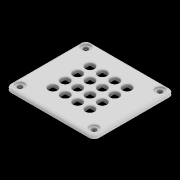
# Autodesk Inventor part: Cubierta Botonera Redonda
Saved by Autodesk Inventor 2020 (Build 240168000, 168)
## iProperties
Created: 2022-02-20
Part Number: Cubierta Botonera Redonda
Material: Genérico
Document SubType Name: Modeling
Designer: Alférez
Density: 1 g/cm^3
Appearance: Valor por defecto
Author: Alférez
Autodesk Inventor part; units mm, degrees
ref_plane "YZ Plane" through (0, 0, 0) normal (1, 0, 0) x (0, 1, 0)
ref_plane "XZ Plane" through (0, 0, 0) normal (0, 1, 0) x (-1, 0, 0)
ref_plane "XY Plane" through (0, 0, 0) normal (0, 0, 1) x (1, 0, 0)
sketch "Boceto1" plane through (0, 0, 0) normal (0, 1, 0) x (-1, 0, 0)
  line L0 (0, 0) -> (90, 0)
  line L1 (90, 0) -> (90, -80)
  line L2 (90, -80) -> (0, -80)
  line L3 (0, -80) -> (0, 0)
  line L4 (0, 0) -> (17, 0)
  line L5 (17, 0) -> (17, -12)
  line L6 (17, -12) -> (28, -12)
  line L7 (28, -12) -> (28, -23)
  line L8 (28, -23) -> (17, -23)
  line L9 (17, -23) -> (17, -12)
  line L10 (17, -23) -> (17, -27)
  line L11 (17, -27) -> (28, -27)
  line L12 (28, -27) -> (28, -38)
  line L13 (28, -38) -> (17, -38)
  line L14 (17, -38) -> (17, -27)
  line L15 (17, -38) -> (17, -42)
  line L16 (17, -42) -> (28, -42)
  line L17 (28, -42) -> (28, -53)
  line L18 (28, -53) -> (17, -53)
  line L19 (17, -53) -> (17, -42)
  line L20 (17, -53) -> (17, -57)
  line L21 (17, -57) -> (28, -57)
  line L22 (28, -57) -> (28, -68)
  line L23 (28, -68) -> (17, -68)
  line L24 (17, -68) -> (17, -57)
  line L25 (32, -12) -> (43, -12)
  line L26 (43, -12) -> (43, -23)
  line L27 (43, -23) -> (32, -23)
  line L28 (32, -23) -> (32, -12)
  line L29 (32, -23) -> (32, -27)
  line L30 (32, -27) -> (43, -27)
  line L31 (43, -27) -> (43, -38)
  line L32 (43, -38) -> (32, -38)
  line L33 (32, -38) -> (32, -27)
  line L34 (32, -38) -> (32, -42)
  line L35 (32, -42) -> (43, -42)
  line L36 (43, -42) -> (43, -53)
  line L37 (43, -53) -> (32, -53)
  line L38 (32, -53) -> (32, -42)
  line L39 (32, -53) -> (32, -57)
  line L40 (32, -57) -> (43, -57)
  line L41 (43, -57) -> (43, -68)
  line L42 (43, -68) -> (32, -68)
  line L43 (32, -68) -> (32, -57)
  line L44 (43, -12) -> (47, -12)
  line L45 (47, -12) -> (58, -12)
  line L46 (58, -12) -> (58, -23)
  line L47 (58, -23) -> (47, -23)
  line L48 (47, -23) -> (47, -12)
  line L49 (47, -23) -> (47, -27)
  line L50 (47, -27) -> (58, -27)
  line L51 (58, -27) -> (58, -38)
  line L52 (58, -38) -> (47, -38)
  line L53 (47, -38) -> (47, -27)
  line L54 (47, -38) -> (47, -42)
  line L55 (47, -42) -> (58, -42)
  line L56 (58, -42) -> (58, -53)
  line L57 (58, -53) -> (47, -53)
  line L58 (47, -53) -> (47, -42)
  line L59 (47, -53) -> (47, -57)
  line L60 (47, -57) -> (58, -57)
  line L61 (58, -57) -> (58, -68)
  line L62 (58, -68) -> (47, -68)
  line L63 (47, -68) -> (47, -57)
  line L64 (58, -12) -> (62, -12)
  line L65 (73, -23) -> (62, -23)
  line L66 (62, -23) -> (62, -27)
  line L67 (62, -27) -> (73, -27)
  line L68 (73, -12) -> (73, -23)
  line L69 (62, -23) -> (62, -12)
  line L70 (62, -38) -> (62, -27)
  line L71 (62, -38) -> (62, -42)
  line L72 (73, -38) -> (62, -38)
  line L73 (73, -27) -> (73, -38)
  line L74 (62, -12) -> (73, -12)
  line L75 (62, -42) -> (73, -42)
  line L76 (62, -53) -> (62, -42)
  line L77 (73, -42) -> (73, -53)
  line L78 (62, -53) -> (62, -57)
  line L79 (62, -57) -> (73, -57)
  line L80 (62, -68) -> (62, -57)
  line L81 (73, -57) -> (73, -68)
  line L82 (73, -68) -> (62, -68)
  line L83 (73, -53) -> (62, -53)
  line L84 (28, -12) -> (32, -12)
  line L85 (0, 0) -> (8.5, 0)
  line L86 (0, 8.5) -> (0, 0)
  line L87 (0, 0) -> (-8.5, 0)
  line L88 (0, -8.5) -> (0, 0)
  line L89 (0, -80) -> (8.5, -80)
  line L90 (0, -88.5) -> (0, -80)
  line L91 (0, -80) -> (-8.5, -80)
  line L92 (0, -71.5) -> (0, -80)
  line L93 (90, 0) -> (81.5, 0)
  line L94 (90, 8.5) -> (90, 0)
  line L95 (90, 0) -> (98.5, 0)
  line L96 (90, -8.5) -> (90, 0)
  line L97 (90, -80) -> (81.5, -80)
  line L98 (81.5, -80) -> (81.5, -71.5)
  line L99 (90, -80) -> (98.5, -80)
  line L100 (90, -71.5) -> (90, -80)
  circle A0 centre (90, 0) radius 3
  circle A1 centre (90, -80) radius 3
  circle A2 centre (0, 0) radius 3
  circle A3 centre (0, -80) radius 3
  line L101 (0, 0) -> (-8.5, 0)
  line L102 (-8.5, 0) -> (-8.5, 8.5)
  line L103 (-8.5, 8.5) -> (0, 8.5)
  line L104 (0, 8.5) -> (0, 0)
  line L105 (0, -88.5) -> (-8.5, -88.5)
  line L106 (-8.5, -88.5) -> (-8.5, -80)
  line L107 (-8.5, -80) -> (0, -80)
  line L108 (0, -80) -> (0, -88.5)
  line L109 (98.5, 0) -> (90, 0)
  line L110 (90, 0) -> (90, 8.5)
  line L111 (90, 8.5) -> (98.5, 8.5)
  line L112 (98.5, 8.5) -> (98.5, 0)
  line L113 (98.5, -88.5) -> (90, -88.5)
  line L114 (90, -88.5) -> (90, -80)
  line L115 (90, -80) -> (98.5, -80)
  line L116 (98.5, -80) -> (98.5, -88.5)
  line L117 (98.5, 8.5) -> (-8.5, 8.5)
  line L118 (-8.5, 8.5) -> (-8.5, -88.5)
  line L119 (-8.5, -88.5) -> (98.5, -88.5)
  line L120 (98.5, -88.5) -> (98.5, 8.5)
  dimension "d0" = 90
  dimension "d1" = 80
  dimension "d2" = 17
  dimension "d3" = 12
  dimension "d4" = 11
  dimension "d5" = 11
  dimension "d6" = 4
  dimension "d7" = 11
  dimension "d8" = 11
  dimension "d9" = 4
  dimension "d10" = 11
  dimension "d11" = 11
  dimension "d12" = 4
  dimension "d13" = 11
  dimension "d14" = 11
  dimension "d16" = 11
  dimension "d17" = 11
  dimension "d18" = 4
  dimension "d19" = 11
  dimension "d20" = 11
  dimension "d21" = 4
  dimension "d22" = 11
  dimension "d23" = 11
  dimension "d24" = 4
  dimension "d25" = 11
  dimension "d26" = 11
  dimension "d27" = 4
  dimension "d28" = 11
  dimension "d29" = 11
  dimension "d30" = 4
  dimension "d31" = 11
  dimension "d32" = 11
  dimension "d33" = 4
  dimension "d34" = 11
  dimension "d35" = 11
  dimension "d36" = 4
  dimension "d37" = 11
  dimension "d38" = 11
  dimension "d39" = 4
  dimension "d40" = 11
  dimension "d41" = 11
  dimension "d42" = 4
  dimension "d43" = 11
  dimension "d44" = 11
  dimension "d45" = 4
  dimension "d46" = 11
  dimension "d47" = 11
  dimension "d48" = 4
  dimension "d49" = 11
  dimension "d50" = 11
  dimension "d51" = 4
  dimension "d52" = 8.5
  dimension "d53" = 8.5
  dimension "d54" = 8.5
  dimension "d55" = 8.5
  dimension "d56" = 8.5
  dimension "d57" = 8.5
  dimension "d58" = 8.5
  dimension "d59" = 6
  dimension "d60" = 6
  dimension "d61" = 6
  dimension "d62" = 8.5
  dimension "d63" = 8.5
  dimension "d64" = 8.5
  constraints: 242 end point, 52 equal length, 29 horizontal, 27 perpendicular, 12 vertical, 4 centre point, 4 coincident, 1 point on line
  measures "d0" distance of L1.end L2.end
  measures "d1" distance of L0.end L1.end
  measures "d2" distance of L0.start L4.end
  measures "d3" distance of L4.end L5.end
  measures "d4" distance of L7.end L8.end
  measures "d5" distance of L6.end L7.end
  measures "d6" distance of L8.end L10.end
  measures "d7" distance of L12.end L13.end
  measures "d8" distance of L11.end L12.end
  measures "d9" distance of L13.end L15.end
  measures "d10" distance of L17.end L18.end
  measures "d11" distance of L16.end L17.end
  measures "d12" distance of L18.end L20.end
  measures "d13" distance of L22.end L23.end
  measures "d14" distance of L21.end L22.end
  measures "d16" distance of L27.start L27.end
  measures "d17" distance of L26.start L27.start
  measures "d18" distance of L27.end L29.end
  measures "d19" distance of L32.start L33.start
  measures "d20" distance of L30.end L32.start
  measures "d21" distance of L33.start L34.end
  measures "d22" distance of L36.end L38.start
  measures "d23" distance of L35.end L36.end
  measures "d24" distance of L38.start L39.end
  measures "d25" distance of L41.end L43.start
  measures "d26" distance of L40.end L41.end
  measures "d27" distance of L26.start L44.end
  measures "d28" distance of L47.start L49.start
  measures "d29" distance of L46.start L47.start
  measures "d30" distance of L49.start L53.end
  measures "d31" distance of L52.start L53.start
  measures "d32" distance of L50.end L52.start
  measures "d33" distance of L53.start L54.end
  measures "d34" distance of L57.start L58.start
  measures "d35" distance of L55.end L57.start
  measures "d36" distance of L58.start L59.end
  measures "d37" distance of L61.end L62.end
  measures "d38" distance of L60.end L61.end
  measures "d39" distance of L46.start L64.end
  measures "d40" distance of L68.end L66.start
  measures "d41" distance of L68.start L68.end
  measures "d42" distance of L66.start L66.end
  measures "d43" distance of L72.start L70.start
  measures "d44" distance of L67.end L72.start
  measures "d45" distance of L70.start L76.end
  measures "d46" distance of L83.start L78.start
  measures "d47" distance of L77.start L83.start
  measures "d48" distance of L78.start L80.end
  measures "d49" distance of L81.end L82.end
  measures "d50" distance of L81.start L81.end
  measures "d51" distance of L6.end L84.end
  measures "d52" distance of L86.end L87.end
  measures "d53" distance of L86.start L86.end
  measures "d54" distance of L91.end L90.end
  measures "d55" distance of L90.end L90.start
  measures "d56" distance of L95.end L94.end
  measures "d57" distance of L94.end L94.start
  measures "d58" distance of L99.start L99.end
  measures "d59" diameter of A0
  measures "d60" diameter of A1
  measures "d61" diameter of A2
  measures "d62" distance of L102.end L103.end
  measures "d63" distance of L101.end L102.end
  measures "d64" distance of L106.end L108.start
extrude "Extrusión1" add sketch "Boceto1" along normal blind 3 contours A2 L86 L117 L94 A0 L0 | L0 A0 L1 A1 L2 A3 L3 A2 | L3 A3 L91 L118 L87 A2 | A2 L87 L102 L103 L86 | L111 L112 L95 A0 L94 | L91 A3 L90 L105 L106 | L2 A1 L114 L119 L90 A3 | L95 L120 L99 A1 L1 A0 | L116 L113 L114 A1 L99
fillet "Empalme1" radius 6 4 edges at (-98.5, 1.5, 8.5) (-98.5, 1.5, -88.5) (8.5, 1.5, 8.5) (8.5, 1.5, -88.5)
fillet "Empalme2" radius 2 16 edges at (-96.7426, 3, -86.7426) (-98.5, 3, 1.25) (-98.5, 3, -40) (-98.5, 3, -81.25) (-96.7426, 3, 6.7426) (1.25, 3, 8.5) (-45, 3, 8.5) (-91.25, 3, 8.5) (6.7426, 3, 6.7426) (8.5, 3, 1.25) (8.5, 3, -40) (8.5, 3, -81.25) (6.7426, 3, -86.7426) (1.25, 3, -88.5) (-45, 3, -88.5) (-91.25, 3, -88.5)
fillet "Empalme3" radius 5.5 63 edges at (-73, 1.5, -12) (-58, 1.5, -12) (-43, 1.5, -12) (-28, 1.5, -12) (-28, 1.5, -27) (-43, 1.5, -27) (-58, 1.5, -27) (-73, 1.5, -27) (-73, 1.5, -42) (-73, 1.5, -57) (-58, 1.5, -42) (-58, 1.5, -57) (-43, 1.5, -57) (-43, 1.5, -42) (-28, 1.5, -42) (-28, 1.5, -57) (-73, 1.5, -23) (-73, 1.5, -38) (-73, 1.5, -68) (-73, 1.5, -53) (-58, 1.5, -68) (-58, 1.5, -53) (-58, 1.5, -38) (-43, 1.5, -38) (-43, 1.5, -68) (-43, 1.5, -53) (-43, 1.5, -23) (-58, 1.5, -23) (-28, 1.5, -23) (-28, 1.5, -38) (-28, 1.5, -53) (-28, 1.5, -68) (-62, 1.5, -68) (-47, 1.5, -68) (-32, 1.5, -68) (-17, 1.5, -68) (-17, 1.5, -53) (-32, 1.5, -53) (-47, 1.5, -53) (-32, 1.5, -38) (-47, 1.5, -38) (-62, 1.5, -38) (-17, 1.5, -38) (-17, 1.5, -23) (-32, 1.5, -23) (-47, 1.5, -23) (-62, 1.5, -23) (-17, 1.5, -57) (-17, 1.5, -42) (-17, 1.5, -27) (-17, 1.5, -12) (-32, 1.5, -12) (-32, 1.5, -27) (-32, 1.5, -42) (-32, 1.5, -57) (-47, 1.5, -27) (-47, 1.5, -12) (-47, 1.5, -42) (-47, 1.5, -57) (-62, 1.5, -57) (-62, 1.5, -42) (-62, 1.5, -27) (-62, 1.5, -12)
fillet "Empalme4" radius 5.5 1 edges at (-62, 1.5, -53)
sketch "Boceto3" plane through (0, 0, 0) normal (0, -1, 0) x (1, 0, 0)
  line L0 (-73, -12) -> (-62, -12)
  line L1 (-62, -12) -> (-62, -23)
  line L2 (-62, -23) -> (-73, -23)
  line L3 (-73, -23) -> (-73, -12)
  line L4 (-73, -27) -> (-62, -27)
  line L5 (-62, -27) -> (-62, -38)
  line L6 (-62, -38) -> (-73, -38)
  line L7 (-73, -38) -> (-73, -27)
  line L8 (-73, -42) -> (-62, -42)
  line L9 (-62, -42) -> (-62, -53)
  line L10 (-62, -53) -> (-73, -53)
  line L11 (-73, -53) -> (-73, -42)
  line L12 (-73, -57) -> (-62, -57)
  line L13 (-62, -57) -> (-62, -68)
  line L14 (-62, -68) -> (-73, -68)
  line L15 (-73, -68) -> (-73, -57)
  line L16 (-47, -23) -> (-58, -23)
  line L17 (-58, -27) -> (-47, -27)
  line L18 (-47, -12) -> (-47, -23)
  line L19 (-58, -23) -> (-58, -12)
  line L20 (-58, -38) -> (-58, -27)
  line L21 (-47, -38) -> (-58, -38)
  line L22 (-47, -27) -> (-47, -38)
  line L23 (-58, -12) -> (-47, -12)
  line L24 (-58, -42) -> (-47, -42)
  line L25 (-58, -53) -> (-58, -42)
  line L26 (-47, -42) -> (-47, -53)
  line L27 (-58, -57) -> (-47, -57)
  line L28 (-58, -68) -> (-58, -57)
  line L29 (-47, -57) -> (-47, -68)
  line L30 (-47, -68) -> (-58, -68)
  line L31 (-47, -53) -> (-58, -53)
  line L32 (-43, -38) -> (-43, -27)
  line L33 (-43, -27) -> (-32, -27)
  line L34 (-32, -23) -> (-43, -23)
  line L35 (-43, -23) -> (-43, -12)
  line L36 (-32, -12) -> (-32, -23)
  line L37 (-28, -23) -> (-28, -12)
  line L38 (-43, -12) -> (-32, -12)
  line L39 (-32, -38) -> (-43, -38)
  line L40 (-43, -42) -> (-32, -42)
  line L41 (-43, -53) -> (-43, -42)
  line L42 (-17, -57) -> (-17, -68)
  line L43 (-17, -68) -> (-28, -68)
  line L44 (-32, -53) -> (-43, -53)
  line L45 (-28, -68) -> (-28, -57)
  line L46 (-43, -57) -> (-32, -57)
  line L47 (-32, -57) -> (-32, -68)
  line L48 (-32, -68) -> (-43, -68)
  line L49 (-43, -68) -> (-43, -57)
  line L50 (-17, -12) -> (-17, -23)
  line L51 (-28, -12) -> (-17, -12)
  line L52 (-17, -23) -> (-28, -23)
  line L53 (-32, -27) -> (-32, -38)
  line L54 (-28, -38) -> (-28, -27)
  line L55 (-28, -27) -> (-17, -27)
  line L56 (-17, -38) -> (-28, -38)
  line L57 (-17, -27) -> (-17, -38)
  line L58 (-28, -57) -> (-17, -57)
  line L59 (-32, -42) -> (-32, -53)
  line L60 (-28, -53) -> (-28, -42)
  line L61 (-17, -53) -> (-28, -53)
  line L62 (-17, -42) -> (-17, -53)
  line L63 (-28, -42) -> (-17, -42)
  circle A0 centre (0, 0) radius 3
  circle A1 centre (0, -80) radius 3
  circle A2 centre (-90, 0) radius 3
  circle A3 centre (-90, -80) radius 3
  line L64 (-98.5, 0) -> (-98.5, 8.5)
  line L65 (-98.5, 8.5) -> (-90, 8.5)
  line L66 (-90, -88.5) -> (-98.5, -88.5)
  line L67 (-98.5, -88.5) -> (-98.5, -80)
  line L68 (8.5, 8.5) -> (8.5, 0)
  line L69 (0, 8.5) -> (8.5, 8.5)
  line L70 (8.5, -80) -> (8.5, -88.5)
  line L71 (8.5, -88.5) -> (0, -88.5)
  line L72 (8.5, 8.5) -> (-98.5, 8.5)
  line L73 (-98.5, 8.5) -> (-98.5, -88.5)
  line L74 (-98.5, -88.5) -> (8.5, -88.5)
  line L75 (8.5, -88.5) -> (8.5, 8.5)
  point P0 (0, 0)
  dimension "d82" = 4
  dimension "d84" = 11
  dimension "d85" = 4
  dimension "d87" = 11
  dimension "d88" = 4
  dimension "d89" = 11
  dimension "d90" = 11
  dimension "d95" = 11
  dimension "d98" = 11
  dimension "d100" = 11
  dimension "d101" = 11
  dimension "d107" = 11
  dimension "d110" = 11
  dimension "d112" = 11
  dimension "d113" = 11
  dimension "d116" = 11
  dimension "d119" = 11
  dimension "d122" = 11
  dimension "d124" = 11
  dimension "d125" = 11
  dimension "d134" = 6
  dimension "d135" = 6
  dimension "d136" = 6
  dimension "d137" = 8.5
  dimension "d138" = 8.5
  dimension "d140" = 8.5
  dimension "d141" = 8.5
  constraints: 152 end point, 34 parallel, 19 horizontal, 18 perpendicular, 4 centre point
  measures "d82" distance of L3.start L7.end
  measures "d84" distance of L5.start L5.end
  measures "d85" distance of L6.end L11.end
  measures "d87" distance of L9.start L9.end
  measures "d88" distance of L10.end L15.end
  measures "d89" distance of L13.end L15.start
  measures "d90" distance of L13.start L13.end
  measures "d95" distance of L22.start L22.end
  measures "d98" distance of L24.end L26.end
  measures "d100" distance of L30.start L30.end
  measures "d101" distance of L27.end L30.start
  measures "d107" distance of L53.start L39.start
  measures "d110" distance of L40.end L44.start
  measures "d112" distance of L47.end L48.end
  measures "d113" distance of L47.start L47.end
  measures "d116" distance of L50.start L52.start
  measures "d119" distance of L57.start L56.start
  measures "d122" distance of L63.end L62.end
  measures "d124" distance of L43.start L45.start
  measures "d125" distance of L42.start L43.start
  measures "d134" diameter of A0
  measures "d135" diameter of A1
  measures "d136" diameter of A2
  measures "d137" distance of L64.end L65.end
  measures "d138" distance of L64.start L64.end
  measures "d140" distance of L74.start L67.end
  measures "d141" distance of L69.start L72.start
extrude "Extrusión2" add sketch "Boceto3" along normal blind 1.5
fillet "Empalme5" radius 6 4 edges at (8.5, -0.75, 8.5) (-98.5, -0.75, 8.5) (-98.5, -0.75, -88.5) (8.5, -0.75, -88.5)
sketch "Boceto4" plane through (0, 3, 0) normal (0, 1, 0) x (1, 0, 0)
  circle A0 centre (0, 0) radius 5.5
  circle A1 centre (-90, 0) radius 3 projected
  circle A2 centre (-90, 0) radius 5.5
  circle A3 centre (0, 80) radius 3 projected
  circle A4 centre (0, 80) radius 5.5
  circle A5 centre (-90, 80) radius 3 projected
  circle A6 centre (-90, 80) radius 5.5
  dimension "d148" = 11
  dimension "d149" = 11
  dimension "d150" = 11
  dimension "d151" = 11
  constraints: 4 centre point, 4 coincident
  measures "d148" diameter of A0
  measures "d149" diameter of A2
  measures "d150" diameter of A4
  measures "d151" diameter of A6
extrude "Extrusión3" cut sketch "Boceto4" against normal blind 1.5 contours A0 | A2 | A4 | A5 | A6
